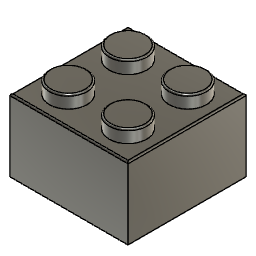
2x2block (Autodesk Fusion 360 design; units mm, degrees)
Autodesk Fusion 360 part; units mm, degrees
sketch "Sketch1" plane through (0, 0, 0) normal (0, 0, 1) x (1, 0, 0)
  line L0 (0, 0) -> (15.8, 0)
  line L1 (15.8, 0) -> (15.8, 15.8)
  line L2 (15.8, 15.8) -> (0, 15.8)
  line L3 (0, 15.8) -> (0, 0)
  constraint coincident L0.start L3.end
extrude "Extrude1" add sketch "Sketch1" along normal blind 9.6
sketch "Sketch2" plane through (0, 0, 9.6) normal (0, 0, 1) x (-1, 0, 0)
  line L0 (0, -15.8) -> (0, 0)
  line L1 (0, 0) -> (-15.8, 0)
  line L2 (-15.8, 0) -> (-15.8, -15.8)
  line L3 (-15.8, -15.8) -> (0, -15.8)
  circle A0 centre (-3.9, -11.9) radius 2.5
extrude "Extrude2" add sketch "Sketch2" along normal blind 1.7 contours A0
pattern_linear "R-Pattern1" count 2 spacing 8 along (1, 0, 0) count 2 spacing 8 along (0, -1, 0) of "Extrude2"
shell "Shell1" thickness 1.49 removed faces 1 at (5.2667, 10.5333, 0)
sketch "Sketch3" plane through (0, 0, 8.11) normal (0, 0, -1) x (1, 0, 0)
  circle A0 centre (11.9, -3.9) radius 1.01
  circle A1 centre (3.9, -3.9) radius 1.01
  circle A2 centre (11.9, -11.9) radius 1.01
  circle A3 centre (3.9, -11.9) radius 1.01
  line L0 (1.49, -1.49) -> (1.49, -14.31)
  line L1 (1.49, -14.31) -> (14.31, -14.31)
  line L2 (14.31, -14.31) -> (14.31, -1.49)
  line L3 (14.31, -1.49) -> (1.49, -1.49)
  circle A4 centre (7.9, -7.9) radius 3.15
  circle A5 centre (7.9, -7.9) radius 2.15
extrude "Extrude3" add sketch "Sketch3" along normal blind 8.1 contours A4
fillet "Fillet1" radius 0.2 8 edges at (6.2308, 12.804, 11.3) (14.2308, 12.804, 11.3) (14.2308, 4.804, 11.3) (6.2308, 4.804, 11.3) (7.9, 0, 9.6) (0, 7.9, 9.6) (15.8, 7.9, 9.6) (7.9, 15.8, 9.6)
scale "Scale1" factor 0.75 about (5.75, 7.9, 8.11) bodies 1
